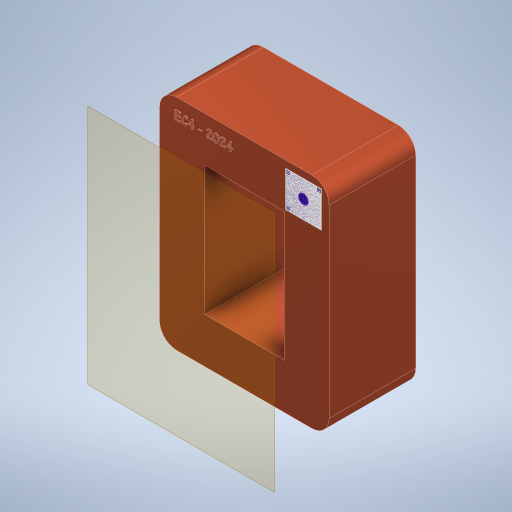
# Autodesk Inventor part: Bobina
Saved by Autodesk Inventor 2024.2 (Build 282272000, 272)
## iProperties
Created: 2024-05-06
Part Number: Bobina
Material: Copper
Document SubType Name: Modeling
Designer: 082220028
Density: 8.94 g/cm^3
Appearance: Copper - Satin
Author: 082220028
Autodesk Inventor part; units mm, degrees
ref_plane "YZ Plane" through (0, 0, 0) normal (1, 0, 0) x (0, 1, 0)
ref_plane "XZ Plane" through (0, 0, 0) normal (0, 1, 0) x (-1, 0, 0)
ref_plane "XY Plane" through (0, 0, 0) normal (0, 0, 1) x (1, 0, 0)
sketch "Sketch1" plane through (0, 0, 0) normal (0, 0, 1) x (1, 0, 0)
  line L0 (0, 0) -> (23, 0)
  line L1 (0, 0) -> (0, 37.338)
  line L2 (0, 37.338) -> (23, 37.338)
  line L3 (23, 37.338) -> (23, 0)
  line L4 (36, -13) -> (-13, -13)
  line L5 (-13, -13) -> (-13, 50.338)
  line L6 (-13, 50.338) -> (36, 50.338)
  line L7 (36, 50.338) -> (36, -13)
  dimension "d0" = 37.338
  dimension "d1" = 23
  dimension "d2" = 13
  constraints: 16 end point, 2 parallel, 2 perpendicular, 1 horizontal, 1 vertical, 3 other
  measures "d0" distance of L2.end L0.end
  measures "d1" distance of L1.end L2.end
  measures "d2" distance between parallel lines of L3 L7
extrude "Extrusion1" add sketch "Sketch1" along normal blind 25
fillet "Fillet1" radius 5 4 edges at (36, 50.338, 12.5) (-13, 50.338, 12.5) (36, -13, 12.5) (-13, -13, 12.5)
ref_plane "Work Plane1" through (0, 0, 55.5) normal (0, 0, 1) x (1, 0, 0)
sketch "Sketch2" plane through (0, 0, 55.5) normal (0, 0, 1) x (1, 0, 0)
  line L0 (23.3211, 48.0815) -> (33.3211, 48.0815) construction
  line L1 (33.3211, 48.0815) -> (33.3211, 38.0815) construction
  line L2 (33.3211, 38.0815) -> (23.3211, 38.0815) construction
  line L3 (23.3211, 38.0815) -> (23.3211, 48.0815) construction
  point P0 (0, 0)
  dimension "d8" = 10
  constraints: 2 other
  measures "d8" distance of L0.start L0.end
decal "Decal1"
ref_plane "Work Plane2" through (0, 0, 49.25) normal (0, 0, 1) x (1, 0, 0)
sketch "Sketch3" plane through (0, 0, 49.25) normal (0, 0, 1) x (1, 0, 0)
  line L0 (-8.6743, 47.2483) -> (12.9355, 47.2483) construction
  line L1 (12.9355, 47.2483) -> (12.9355, 43.4488) construction
  line L2 (12.9355, 43.4488) -> (-8.6743, 43.4488) construction
  line L3 (-8.6743, 43.4488) -> (-8.6743, 47.2483) construction
  spline S0 degree 2 poles (-6.9225, 46.841) (-6.9444, 46.841) (-6.9729, 46.8498) knots 0 0 0 1 1 1
  spline S1 degree 2 poles (-6.9729, 46.8498) (-7.2378, 46.9242) (-7.4853, 46.9242) knots 0 0 0 1 1 1
  spline S2 degree 2 poles (-7.4853, 46.9242) (-7.6123, 46.9242) (-7.9188, 46.8782) (-8.094, 46.8301) knots 0 0 0 1 2 2 2
  spline S3 degree 2 poles (-8.094, 46.8301) (-8.0787, 46.7271) (-8.0787, 46.6658) knots 0 0 0 1 1 1
  spline S4 degree 2 poles (-8.0787, 46.6658) (-8.0787, 46.4491) (-8.1071, 46.0659) knots 0 0 0 1 1 1
  line L4 (-8.1071, 46.0659) -> (-7.4174, 46.1316)
  spline S5 degree 2 poles (-7.4174, 46.1316) (-7.1152, 46.1622) (-7.0473, 46.1622) knots 0 0 0 1 1 1
  spline S6 degree 2 poles (-7.0473, 46.1622) (-6.9773, 46.1622) (-6.8831, 46.0746) (-6.8831, 46.0002) knots 0 0 0 1 2 2 2
  spline S7 degree 2 poles (-6.8831, 46.0002) (-6.8831, 45.8579) (-7.0276, 45.8403) knots 0 0 0 1 1 1
  line L5 (-7.0276, 45.8403) -> (-7.4021, 45.8075)
  line L6 (-7.4021, 45.8075) -> (-8.129, 45.7418)
  spline S8 degree 2 poles (-8.129, 45.7418) (-8.1356, 45.6301) (-8.1422, 45.4309) (-8.1422, 45.3455) knots 0 0 0 1 2 2 2
  spline S9 degree 2 poles (-8.1422, 45.3455) (-8.1422, 44.9973) (-8.0918, 44.936) knots 0 0 0 1 1 1
  spline S10 degree 2 poles (-8.0918, 44.936) (-8.0546, 44.8922) (-7.8444, 44.8922) knots 0 0 0 1 1 1
  spline S11 degree 2 poles (-7.8444, 44.8922) (-7.748, 44.8922) (-7.3561, 44.9032) (-7.2576, 44.9032) knots 0 0 0 1 2 2 2
  spline S12 degree 2 poles (-7.2576, 44.9032) (-7.2269, 44.9032) (-7.1043, 44.9229) (-7.0736, 44.9229) knots 0 0 0 1 2 2 2
  spline S13 degree 2 poles (-7.0736, 44.9229) (-6.9072, 44.9229) (-6.9072, 44.7608) knots 0 0 0 1 1 1
  spline S14 degree 2 poles (-6.9072, 44.7608) (-6.9072, 44.6295) (-7.0408, 44.6032) knots 0 0 0 1 1 1
  spline S15 degree 2 poles (-7.0408, 44.6032) (-7.1875, 44.5725) (-7.6802, 44.5725) knots 0 0 0 1 1 1
  spline S16 degree 2 poles (-7.6802, 44.5725) (-8.1663, 44.5725) (-8.3042, 44.7017) knots 0 0 0 1 1 1
  spline S17 degree 2 poles (-8.3042, 44.7017) (-8.4553, 44.8419) (-8.4553, 45.3455) knots 0 0 0 1 1 1
  spline S18 degree 2 poles (-8.4553, 45.3455) (-8.4553, 45.4462) (-8.4465, 45.6849) (-8.4378, 45.8228) knots 0 0 0 1 2 2 2
  spline S19 degree 2 poles (-8.4378, 45.8228) (-8.4553, 45.8579) (-8.4553, 45.8995) knots 0 0 0 1 1 1
  spline S20 degree 2 poles (-8.4553, 45.8995) (-8.4553, 45.952) (-8.4246, 45.9958) knots 0 0 0 1 1 1
  spline S21 degree 2 poles (-8.4246, 45.9958) (-8.394, 46.4491) (-8.394, 46.6658) knots 0 0 0 1 1 1
  spline S22 degree 2 poles (-8.394, 46.6658) (-8.394, 46.725) (-8.4246, 46.9483) (-8.4246, 47.0074) knots 0 0 0 1 2 2 2
  spline S23 degree 2 poles (-8.4246, 47.0074) (-8.4246, 47.1935) (-8.267, 47.1935) knots 0 0 0 1 1 1
  spline S24 degree 2 poles (-8.267, 47.1935) (-8.2013, 47.1935) (-8.1553, 47.1476) knots 0 0 0 1 1 1
  spline S25 degree 2 poles (-8.1553, 47.1476) (-7.967, 47.1979) (-7.632, 47.2483) (-7.4831, 47.2483) knots 0 0 0 1 2 2 2
  spline S26 degree 2 poles (-7.4831, 47.2483) (-7.1021, 47.2483) (-6.8744, 47.1563) knots 0 0 0 1 1 1
  spline S27 degree 2 poles (-6.8744, 47.1563) (-6.7693, 47.1147) (-6.7693, 47.0052) knots 0 0 0 1 1 1
  spline S28 degree 2 poles (-6.7693, 47.0052) (-6.7693, 46.9439) (-6.8109, 46.8936) knots 0 0 0 1 1 1
  spline S29 degree 2 poles (-6.8109, 46.8936) (-6.8547, 46.841) (-6.9225, 46.841) knots 0 0 0 1 1 1
  spline S30 degree 2 poles (-4.9321, 46.4885) (-5.0329, 46.4885) (-5.0832, 46.6067) knots 0 0 0 1 1 1
  spline S31 degree 2 poles (-5.0832, 46.6067) (-5.127, 46.7074) (-5.1642, 46.7293) knots 0 0 0 1 1 1
  spline S32 degree 2 poles (-5.1642, 46.7293) (-5.1971, 46.7469) (-5.3285, 46.7469) knots 0 0 0 1 1 1
  spline S33 degree 2 poles (-5.3285, 46.7469) (-5.5562, 46.7469) (-5.8343, 46.3987) knots 0 0 0 1 1 1
  spline S34 degree 2 poles (-5.8343, 46.3987) (-6.2109, 45.9301) (-6.2109, 45.5119) knots 0 0 0 1 1 1
  spline S35 degree 2 poles (-6.2109, 45.5119) (-6.2109, 45.3082) (-6.0795, 45.1637) knots 0 0 0 1 1 1
  spline S36 degree 2 poles (-6.0795, 45.1637) (-5.946, 45.0126) (-5.7576, 45.0126) knots 0 0 0 1 1 1
  spline S37 degree 2 poles (-5.7576, 45.0126) (-5.5956, 45.0126) (-5.4336, 45.0959) knots 0 0 0 1 1 1
  spline S38 degree 2 poles (-5.4336, 45.0959) (-5.3416, 45.144) (-5.1533, 45.282) knots 0 0 0 1 1 1
  spline S39 degree 2 poles (-5.1533, 45.282) (-5.0635, 45.3477) (-5.0175, 45.3477) knots 0 0 0 1 1 1
  spline S40 degree 2 poles (-5.0175, 45.3477) (-4.9518, 45.3477) (-4.8599, 45.2447) (-4.8599, 45.1834) knots 0 0 0 1 2 2 2
  spline S41 degree 2 poles (-4.8599, 45.1834) (-4.8599, 45.1112) (-4.919, 45.0586) knots 0 0 0 1 1 1
  spline S42 degree 2 poles (-4.919, 45.0586) (-5.335, 44.6908) (-5.7576, 44.6908) knots 0 0 0 1 1 1
  spline S43 degree 2 poles (-5.7576, 44.6908) (-6.0839, 44.6908) (-6.3072, 44.9404) knots 0 0 0 1 1 1
  spline S44 degree 2 poles (-6.3072, 44.9404) (-6.524, 45.1812) (-6.524, 45.5119) knots 0 0 0 1 1 1
  spline S45 degree 2 poles (-6.524, 45.5119) (-6.524, 46.044) (-6.0773, 46.6023) knots 0 0 0 1 1 1
  spline S46 degree 2 poles (-6.0773, 46.6023) (-5.7051, 47.0687) (-5.3285, 47.0687) knots 0 0 0 1 1 1
  spline S47 degree 2 poles (-5.3285, 47.0687) (-5.2518, 47.0687) (-5.1292, 47.0556) (-5.081, 47.0381) knots 0 0 0 1 2 2 2
  spline S48 degree 2 poles (-5.081, 47.0381) (-5.0263, 47.1191) (-4.9387, 47.1191) knots 0 0 0 1 1 1
  spline S49 degree 2 poles (-4.9387, 47.1191) (-4.8292, 47.1191) (-4.8008, 46.9768) knots 0 0 0 1 1 1
  spline S50 degree 2 poles (-4.8008, 46.9768) (-4.7767, 46.8476) (-4.7767, 46.6636) knots 0 0 0 1 1 1
  spline S51 degree 2 poles (-4.7767, 46.6636) (-4.7767, 46.598) (-4.8117, 46.5498) knots 0 0 0 1 1 1
  spline S52 degree 2 poles (-4.8117, 46.5498) (-4.8533, 46.4885) (-4.9321, 46.4885) knots 0 0 0 1 1 1
  line L7 (-3.2133, 45.4134) -> (-3.2133, 44.8331)
  spline S53 degree 2 poles (-3.2133, 44.8331) (-3.2133, 44.6864) (-3.3556, 44.6864) knots 0 0 0 1 1 1
  spline S54 degree 2 poles (-3.3556, 44.6864) (-3.522, 44.6864) (-3.522, 44.9141) knots 0 0 0 1 1 1
  spline S55 degree 2 poles (-3.522, 44.9141) (-3.522, 44.9426) (-3.5154, 45.0455) (-3.5154, 45.0652) knots 0 0 0 1 2 2 2
  line L8 (-3.5154, 45.0652) -> (-3.5176, 45.4221)
  line L9 (-3.5176, 45.4221) -> (-4.2096, 45.4396)
  spline S56 degree 2 poles (-4.2096, 45.4396) (-4.4263, 45.4396) (-4.5095, 45.4528) knots 0 0 0 1 1 1
  spline S57 degree 2 poles (-4.5095, 45.4528) (-4.6519, 45.4769) (-4.6519, 45.5644) knots 0 0 0 1 1 1
  spline S58 degree 2 poles (-4.6519, 45.5644) (-4.6519, 45.6345) (-4.5665, 45.744) knots 0 0 0 1 1 1
  line L10 (-4.5665, 45.744) -> (-4.4307, 45.9038)
  line L11 (-4.4307, 45.9038) -> (-3.6578, 47.0315)
  spline S59 degree 2 poles (-3.6578, 47.0315) (-3.5527, 47.1782) (-3.3906, 47.1782) knots 0 0 0 1 1 1
  spline S60 degree 2 poles (-3.3906, 47.1782) (-3.2133, 47.1782) (-3.2133, 47.0249) knots 0 0 0 1 1 1
  line L12 (-3.2133, 47.0249) -> (-3.2133, 45.7177)
  spline S61 degree 2 poles (-3.2133, 45.7177) (-3.187, 45.7199) (-3.1498, 45.7199) knots 0 0 0 1 1 1
  spline S62 degree 2 poles (-3.1498, 45.7199) (-2.8607, 45.7199) (-2.8607, 45.5644) knots 0 0 0 1 1 1
  spline S63 degree 2 poles (-2.8607, 45.5644) (-2.8607, 45.4506) (-2.979, 45.4221) knots 0 0 0 1 1 1
  spline S64 degree 2 poles (-2.979, 45.4221) (-3.0337, 45.4068) (-3.2133, 45.4134) knots 0 0 0 1 1 1
  spline S65 degree 2 poles (-3.5176, 46.7447) (-3.9358, 46.0724) (-4.1723, 45.7396) knots 0 0 0 1 1 1
  line L13 (-4.1723, 45.7396) -> (-3.5176, 45.7243)
  line L14 (-3.5176, 45.7243) -> (-3.5176, 46.7447)
  spline S66 degree 2 poles (-0.7368, 45.4747) (-0.9492, 45.4528) (-1.4966, 45.4528) knots 0 0 0 1 1 1
  spline S67 degree 2 poles (-1.4966, 45.4528) (-1.628, 45.4528) (-1.628, 45.5754) knots 0 0 0 1 1 1
  spline S68 degree 2 poles (-1.628, 45.5754) (-1.628, 45.698) (-1.4966, 45.698) knots 0 0 0 1 1 1
  spline S69 degree 2 poles (-1.4966, 45.698) (-1.3718, 45.698) (-0.8747, 45.7199) (-0.7521, 45.7199) knots 0 0 0 1 2 2 2
  spline S70 degree 2 poles (-0.7521, 45.7199) (-0.612, 45.7199) (-0.612, 45.5973) knots 0 0 0 1 1 1
  spline S71 degree 2 poles (-0.612, 45.5973) (-0.612, 45.49) (-0.7368, 45.4747) knots 0 0 0 1 1 1
  spline S72 degree 2 poles (2.0813, 44.7258) (2.0419, 44.7258) (1.8996, 44.774) (1.8602, 44.774) knots 0 0 0 1 2 2 2
  spline S73 degree 2 poles (1.8602, 44.774) (1.7813, 44.774) (1.4617, 44.7543) (1.3784, 44.7543) knots 0 0 0 1 2 2 2
  spline S74 degree 2 poles (1.3784, 44.7543) (1.3171, 44.7543) (1.0785, 44.7236) (1.0172, 44.7236) knots 0 0 0 1 2 2 2
  spline S75 degree 2 poles (1.0172, 44.7236) (0.9996, 44.7236) (0.9339, 44.7367) (0.9164, 44.7367) knots 0 0 0 1 2 2 2
  spline S76 degree 2 poles (0.9164, 44.7367) (0.8091, 44.7367) (0.7763, 44.8419) knots 0 0 0 1 1 1
  spline S77 degree 2 poles (0.7763, 44.8419) (0.7566, 44.8966) (0.7566, 45.0302) knots 0 0 0 1 1 1
  spline S78 degree 2 poles (0.7566, 45.0302) (0.7566, 45.3958) (0.9558, 45.6192) knots 0 0 0 1 1 1
  spline S79 degree 2 poles (0.9558, 45.6192) (1.0478, 45.7199) (1.4463, 45.9958) knots 0 0 0 1 1 1
  spline S80 degree 2 poles (1.4463, 45.9958) (1.6719, 46.1491) (1.7463, 46.2367) knots 0 0 0 1 1 1
  spline S81 degree 2 poles (1.7463, 46.2367) (1.8821, 46.3856) (1.8821, 46.5892) knots 0 0 0 1 1 1
  spline S82 degree 2 poles (1.8821, 46.5892) (1.8821, 46.6899) (1.7529, 46.7687) knots 0 0 0 1 1 1
  spline S83 degree 2 poles (1.7529, 46.7687) (1.6368, 46.8388) (1.5273, 46.8388) knots 0 0 0 1 1 1
  spline S84 degree 2 poles (1.5273, 46.8388) (1.3828, 46.8388) (1.2536, 46.7556) knots 0 0 0 1 1 1
  line L15 (1.2536, 46.7556) -> (1.0281, 46.5782)
  spline S85 degree 2 poles (1.0281, 46.5782) (0.9602, 46.5257) (0.9208, 46.5257) knots 0 0 0 1 1 1
  spline S86 degree 2 poles (0.9208, 46.5257) (0.7588, 46.5257) (0.7588, 46.6549) knots 0 0 0 1 1 1
  spline S87 degree 2 poles (0.7588, 46.6549) (0.7588, 46.7293) (0.8179, 46.7819) knots 0 0 0 1 1 1
  spline S88 degree 2 poles (0.8179, 46.7819) (1.0018, 46.9549) (1.1376, 47.0315) knots 0 0 0 1 1 1
  spline S89 degree 2 poles (1.1376, 47.0315) (1.3259, 47.141) (1.5273, 47.141) knots 0 0 0 1 1 1
  spline S90 degree 2 poles (1.5273, 47.141) (1.7813, 47.141) (1.9806, 47.003) knots 0 0 0 1 1 1
  spline S91 degree 2 poles (1.9806, 47.003) (2.2039, 46.8476) (2.2039, 46.6045) knots 0 0 0 1 1 1
  spline S92 degree 2 poles (2.2039, 46.6045) (2.2039, 46.4425) (2.112, 46.1732) (2.02, 46.0615) knots 0 0 0 1 2 2 2
  spline S93 degree 2 poles (2.02, 46.0615) (1.9018, 45.9192) (1.6215, 45.7462) knots 0 0 0 1 1 1
  spline S94 degree 2 poles (1.6215, 45.7462) (1.3259, 45.5601) (1.2339, 45.4637) knots 0 0 0 1 1 1
  spline S95 degree 2 poles (1.2339, 45.4637) (1.0609, 45.2842) (1.0631, 45.0258) knots 0 0 0 1 1 1
  line L16 (1.0631, 45.0258) -> (1.3872, 45.0542)
  spline S96 degree 2 poles (1.3872, 45.0542) (1.7178, 45.074) (1.8602, 45.074) knots 0 0 0 1 1 1
  spline S97 degree 2 poles (1.8602, 45.074) (1.9806, 45.074) (2.0879, 45.0324) knots 0 0 0 1 1 1
  spline S98 degree 2 poles (2.0879, 45.0324) (2.228, 44.9798) (2.228, 44.8813) knots 0 0 0 1 1 1
  spline S99 degree 2 poles (2.228, 44.8813) (2.228, 44.8221) (2.1426, 44.7258) (2.0813, 44.7258) knots 0 0 0 1 2 2 2
  spline S100 degree 2 poles (3.4236, 44.6667) (2.9462, 44.6667) (2.7273, 45.1024) knots 0 0 0 1 1 1
  spline S101 degree 2 poles (2.7273, 45.1024) (2.5609, 45.4396) (2.5609, 45.9783) knots 0 0 0 1 1 1
  spline S102 degree 2 poles (2.5609, 45.9783) (2.5609, 46.4337) (2.7776, 46.7731) knots 0 0 0 1 1 1
  spline S103 degree 2 poles (2.7776, 46.7731) (3.0338, 47.1695) (3.4718, 47.1695) knots 0 0 0 1 1 1
  spline S104 degree 2 poles (3.4718, 47.1695) (3.8856, 47.1695) (4.1155, 46.8169) knots 0 0 0 1 1 1
  spline S105 degree 2 poles (4.1155, 46.8169) (4.3148, 46.5126) (4.3148, 46.0746) knots 0 0 0 1 1 1
  spline S106 degree 2 poles (4.3148, 46.0746) (4.3148, 45.3717) (3.8703, 44.6667) (3.4236, 44.6667) knots 0 0 0 1 2 2 2
  spline S107 degree 2 poles (3.4718, 46.8673) (3.1783, 46.8673) (3.0075, 46.5695) knots 0 0 0 1 1 1
  spline S108 degree 2 poles (3.0075, 46.5695) (2.8652, 46.3221) (2.8652, 46.0046) knots 0 0 0 1 1 1
  spline S109 degree 2 poles (2.8652, 46.0046) (2.8652, 45.4878) (3.1455, 44.9689) (3.4236, 44.9689) knots 0 0 0 1 2 2 2
  spline S110 degree 2 poles (3.4236, 44.9689) (3.7564, 44.9689) (3.9009, 45.3499) knots 0 0 0 1 1 1
  spline S111 degree 2 poles (3.9009, 45.3499) (4.0017, 45.6126) (4.0017, 46.0177) knots 0 0 0 1 1 1
  spline S112 degree 2 poles (4.0017, 46.0177) (4.0017, 46.4425) (3.7367, 46.8673) (3.4718, 46.8673) knots 0 0 0 1 2 2 2
  spline S113 degree 2 poles (6.0096, 44.7258) (5.9702, 44.7258) (5.8278, 44.774) (5.7884, 44.774) knots 0 0 0 1 2 2 2
  spline S114 degree 2 poles (5.7884, 44.774) (5.7096, 44.774) (5.3899, 44.7543) (5.3067, 44.7543) knots 0 0 0 1 2 2 2
  spline S115 degree 2 poles (5.3067, 44.7543) (5.2454, 44.7543) (5.0067, 44.7236) (4.9454, 44.7236) knots 0 0 0 1 2 2 2
  spline S116 degree 2 poles (4.9454, 44.7236) (4.9279, 44.7236) (4.8622, 44.7367) (4.8447, 44.7367) knots 0 0 0 1 2 2 2
  spline S117 degree 2 poles (4.8447, 44.7367) (4.7374, 44.7367) (4.7045, 44.8419) knots 0 0 0 1 1 1
  spline S118 degree 2 poles (4.7045, 44.8419) (4.6848, 44.8966) (4.6848, 45.0302) knots 0 0 0 1 1 1
  spline S119 degree 2 poles (4.6848, 45.0302) (4.6848, 45.3958) (4.8841, 45.6192) knots 0 0 0 1 1 1
  spline S120 degree 2 poles (4.8841, 45.6192) (4.976, 45.7199) (5.3746, 45.9958) knots 0 0 0 1 1 1
  spline S121 degree 2 poles (5.3746, 45.9958) (5.6001, 46.1491) (5.6745, 46.2367) knots 0 0 0 1 1 1
  spline S122 degree 2 poles (5.6745, 46.2367) (5.8103, 46.3856) (5.8103, 46.5892) knots 0 0 0 1 1 1
  spline S123 degree 2 poles (5.8103, 46.5892) (5.8103, 46.6899) (5.6811, 46.7687) knots 0 0 0 1 1 1
  spline S124 degree 2 poles (5.6811, 46.7687) (5.5651, 46.8388) (5.4556, 46.8388) knots 0 0 0 1 1 1
  spline S125 degree 2 poles (5.4556, 46.8388) (5.3111, 46.8388) (5.1819, 46.7556) knots 0 0 0 1 1 1
  line L17 (5.1819, 46.7556) -> (4.9563, 46.5782)
  spline S126 degree 2 poles (4.9563, 46.5782) (4.8885, 46.5257) (4.849, 46.5257) knots 0 0 0 1 1 1
  spline S127 degree 2 poles (4.849, 46.5257) (4.687, 46.5257) (4.687, 46.6549) knots 0 0 0 1 1 1
  spline S128 degree 2 poles (4.687, 46.6549) (4.687, 46.7293) (4.7461, 46.7819) knots 0 0 0 1 1 1
  spline S129 degree 2 poles (4.7461, 46.7819) (4.9301, 46.9549) (5.0658, 47.0315) knots 0 0 0 1 1 1
  spline S130 degree 2 poles (5.0658, 47.0315) (5.2541, 47.141) (5.4556, 47.141) knots 0 0 0 1 1 1
  spline S131 degree 2 poles (5.4556, 47.141) (5.7096, 47.141) (5.9088, 47.003) knots 0 0 0 1 1 1
  spline S132 degree 2 poles (5.9088, 47.003) (6.1322, 46.8476) (6.1322, 46.6045) knots 0 0 0 1 1 1
  spline S133 degree 2 poles (6.1322, 46.6045) (6.1322, 46.4425) (6.0402, 46.1732) (5.9483, 46.0615) knots 0 0 0 1 2 2 2
  spline S134 degree 2 poles (5.9483, 46.0615) (5.83, 45.9192) (5.5497, 45.7462) knots 0 0 0 1 1 1
  spline S135 degree 2 poles (5.5497, 45.7462) (5.2541, 45.5601) (5.1622, 45.4637) knots 0 0 0 1 1 1
  spline S136 degree 2 poles (5.1622, 45.4637) (4.9892, 45.2842) (4.9914, 45.0258) knots 0 0 0 1 1 1
  line L18 (4.9914, 45.0258) -> (5.3154, 45.0542)
  spline S137 degree 2 poles (5.3154, 45.0542) (5.6461, 45.074) (5.7884, 45.074) knots 0 0 0 1 1 1
  spline S138 degree 2 poles (5.7884, 45.074) (5.9088, 45.074) (6.0161, 45.0324) knots 0 0 0 1 1 1
  spline S139 degree 2 poles (6.0161, 45.0324) (6.1563, 44.9798) (6.1563, 44.8813) knots 0 0 0 1 1 1
  spline S140 degree 2 poles (6.1563, 44.8813) (6.1563, 44.8221) (6.0709, 44.7258) (6.0096, 44.7258) knots 0 0 0 1 2 2 2
  line L19 (7.9058, 45.4134) -> (7.9058, 44.8331)
  spline S141 degree 2 poles (7.9058, 44.8331) (7.9058, 44.6864) (7.7635, 44.6864) knots 0 0 0 1 1 1
  spline S142 degree 2 poles (7.7635, 44.6864) (7.5971, 44.6864) (7.5971, 44.9141) knots 0 0 0 1 1 1
  spline S143 degree 2 poles (7.5971, 44.9141) (7.5971, 44.9426) (7.6036, 45.0455) (7.6036, 45.0652) knots 0 0 0 1 2 2 2
  line L20 (7.6036, 45.0652) -> (7.6014, 45.4221)
  line L21 (7.6014, 45.4221) -> (6.9095, 45.4396)
  spline S144 degree 2 poles (6.9095, 45.4396) (6.6927, 45.4396) (6.6095, 45.4528) knots 0 0 0 1 1 1
  spline S145 degree 2 poles (6.6095, 45.4528) (6.4672, 45.4769) (6.4672, 45.5644) knots 0 0 0 1 1 1
  spline S146 degree 2 poles (6.4672, 45.5644) (6.4672, 45.6345) (6.5526, 45.744) knots 0 0 0 1 1 1
  line L22 (6.5526, 45.744) -> (6.6884, 45.9038)
  line L23 (6.6884, 45.9038) -> (7.4613, 47.0315)
  spline S147 degree 2 poles (7.4613, 47.0315) (7.5664, 47.1782) (7.7284, 47.1782) knots 0 0 0 1 1 1
  spline S148 degree 2 poles (7.7284, 47.1782) (7.9058, 47.1782) (7.9058, 47.0249) knots 0 0 0 1 1 1
  line L24 (7.9058, 47.0249) -> (7.9058, 45.7177)
  spline S149 degree 2 poles (7.9058, 45.7177) (7.9321, 45.7199) (7.9693, 45.7199) knots 0 0 0 1 1 1
  spline S150 degree 2 poles (7.9693, 45.7199) (8.2583, 45.7199) (8.2583, 45.5644) knots 0 0 0 1 1 1
  spline S151 degree 2 poles (8.2583, 45.5644) (8.2583, 45.4506) (8.1401, 45.4221) knots 0 0 0 1 1 1
  spline S152 degree 2 poles (8.1401, 45.4221) (8.0854, 45.4068) (7.9058, 45.4134) knots 0 0 0 1 1 1
  spline S153 degree 2 poles (7.6014, 46.7447) (7.1832, 46.0724) (6.9467, 45.7396) knots 0 0 0 1 1 1
  line L25 (6.9467, 45.7396) -> (7.6014, 45.7243)
  line L26 (7.6014, 45.7243) -> (7.6014, 46.7447)
  point P0 (0, 0)
  constraints: 2 other
emboss "Emboss1" sketch "Sketch3" operation add depth 0.3 direction (0, 0, -1)
ref_plane "Work Plane3" through (0, 0, 43.25) normal (0, 0, 1) x (1, 0, 0)
sketch "Sketch4" plane through (0, 0, 43.25) normal (0, 0, 1) x (1, 0, 0)
  line L0 (23.307, 48.3528) -> (33.807, 48.3528) construction
  line L1 (33.807, 48.3528) -> (33.807, 37.8528) construction
  line L2 (33.807, 37.8528) -> (23.307, 37.8528) construction
  line L3 (23.307, 37.8528) -> (23.307, 48.3528) construction
  point P0 (0, 0)
  dimension "d25" = 10.5
  constraints: 2 other
  measures "d25" distance of L0.start L0.end
decal "Decal2"
body "Solid1"
